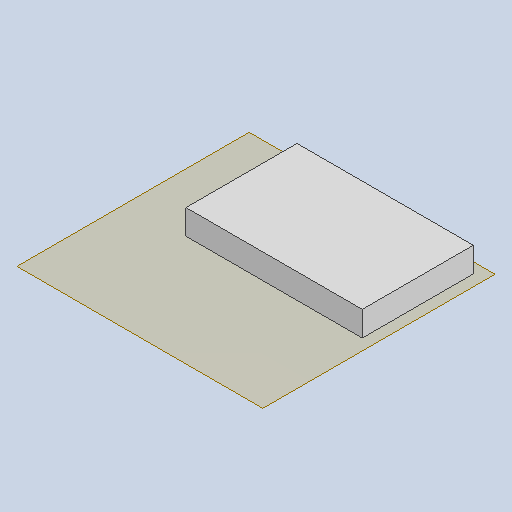
# Autodesk Inventor part: каретка
Saved by Autodesk Inventor 2024.2 (Build 282272000, 272)
## iProperties
Created: 2026-02-13
Part Number: каретка
Material: Типовые
Document SubType Name: Modeling
Designer: Service
Density: 1 g/cm^3
Appearance: По умолчанию
Author: Service
Autodesk Inventor part; units mm, degrees
ref_plane "YZ Plane" through (0, 0, 0) normal (1, 0, 0) x (0, 1, 0)
ref_plane "XZ Plane" through (0, 0, 0) normal (0, 1, 0) x (-1, 0, 0)
ref_plane "XY Plane" through (0, 0, 0) normal (0, 0, 1) x (1, 0, 0)
ref_plane "РабПлоскость1" through (-7.5749, -280.0826, 223.3085) normal (0, 1, 0) x (-1, 0, 0)
sketch "Эскиз1" plane through (-7.5749, -280.0826, 223.3085) normal (0, 1, 0) x (-1, 0, 0)
  line L0 (14.1968, 2.6473) -> (0, 2.6473)
  line L1 (0, 2.6473) -> (0, -6.2943)
  line L2 (0, -6.2943) -> (14.1968, -6.2943)
  line L3 (14.1968, -6.2943) -> (14.1968, 2.6473)
  line L4 (4.1714, -6.2943) -> (16.1714, -6.2943) projected
  line L5 (0, -6.2943) -> (0, 0) projected
  circle A0 centre (9.1714, -1.5852) radius 2.75 projected
  point P0 (-7.5749, -223.3085)
  point P1 (6.5045, -0.9144)
  point P2 (6.5045, -2.256)
  constraints: 8 end point, 2 collinear, 2 parallel, 1 horizontal, 1 perpendicular
extrude "Выдавливание1" add sketch "Эскиз1" along normal blind 2 contours L3 L2 L1 L0 | A0
